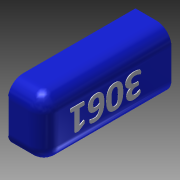
# Autodesk Inventor part: Bumper Cover Part4 (24x28 robot)
Saved by Autodesk Inventor 2013 (Build 170138000, 138)
## iProperties
Created: 2013-01-06
Part Number: Bumper Cover Part4 (24x28 robot)
Material: Generic
Document SubType Name: Modeling
Designer: Moses
Density: 1 g/cm^3
Mass: 165.217 g
Surface Area: 2027.83 cm^2
Volume: 165.217 cm^3
Author: Moses
Autodesk Inventor part; units mm, degrees
ref_plane "YZ Plane" through (0, 0, 0) normal (1, 0, 0) x (0, 1, 0)
ref_plane "XZ Plane" through (0, 0, 0) normal (0, 1, 0) x (-1, 0, 0)
ref_plane "XY Plane" through (0, 0, 0) normal (0, 0, 1) x (1, 0, 0)
sketch "Sketch1" plane through (0, 0, 0) normal (0, 0, 1) x (1, 0, 0)
  line L0 (-6.35, 63.5) -> (-6.35, -63.5) construction
  line L1 (6.35, 63.5) -> (-6.35, 63.5) construction
  line L2 (-6.35, -63.5) -> (6.35, -63.5) construction
  circle A0 centre (38.1, -31.75) radius 31.75 construction
  circle A1 centre (38.1, 31.75) radius 31.75 construction
  line L3 (6.35, 63.5) -> (38.1, 63.5) construction
  line L4 (69.85, 31.75) -> (69.85, -31.75) construction
  line L5 (6.35, -63.5) -> (38.1, -63.5) construction
  line L6 (38.1, 65.0875) -> (-7.9375, 65.0875)
  line L7 (-7.9375, -65.0875) -> (38.1, -65.0875)
  arc A2 (38.1, -65.0875) -> (71.4375, -31.75) centre (38.1, -31.75) ccw
  arc A3 (71.4375, 31.75) -> (38.1, 65.0875) centre (38.1, 31.75) ccw
  line L8 (71.4375, 31.75) -> (71.4375, -31.75)
  line L9 (38.1, 65.0875) -> (38.1, 63.5) construction
  arc A4 (69.85, 31.75) -> (38.1, 63.5) centre (38.1, 31.75) ccw
  arc A5 (38.1, -63.5) -> (69.85, -31.75) centre (38.1, -31.75) ccw
  line L10 (38.1, 63.5) -> (-6.35, 63.5)
  line L11 (38.1, -63.5) -> (-6.35, -63.5)
  line L12 (69.85, 31.75) -> (69.85, -31.75)
  line L13 (-6.35, 63.5) -> (-6.35, 38.1)
  line L14 (-6.35, 38.1) -> (-7.9375, 38.1)
  line L15 (-7.9375, 38.1) -> (-7.9375, 65.0875)
  line L16 (-7.9375, -65.0875) -> (-7.9375, -38.1)
  line L17 (-7.9375, -38.1) -> (-6.35, -38.1)
  line L18 (-6.35, -63.5) -> (-6.35, -38.1)
  line L19 (-6.35, 38.1) -> (-6.35, -38.1)
  point P0 (0, 0)
  point P1 (38.1, 64.2937)
  dimension "d3" = 25.4
  dimension "d5" = 1.5875
  dimension "d6" = 1.5875
  dimension "d7" = 25.4
  dimension "d9" = 1.5875
  constraints: 34 end point, 14 tangent, 12 point on circle, 6 perpendicular, 4 centre point, 3 collinear, 3 parallel, 2 coincident, 2 point on line, 1 concentric, 1 midpoint, 1 vertical
  measures "d3" distance of L0.start L13.end
  measures "d5" distance between parallel lines of L0 L15
  measures "d6" distance between parallel lines of L0 L16
  measures "d7" distance of L0.end L17.end
  measures "d9" distance of L6.start L3.end
extrude "Extrusion1" add sketch "Sketch1" along normal blind 1.5875
extrude "Extrusion2" add sketch "Sketch1" against normal blind 277.8125 contours A3 L8 A2 L7 L16 L17 L18 L11 A5 L12 A4 L10 L13 L14 L15 L6
sketch "Sketch2" plane through (0, 0, -277.8125) normal (0, 0, -1) x (-1, 0, 0)
  line L0 (-38.1, 63.5) -> (6.35, 63.5) projected
  line L1 (6.35, 63.5) -> (6.35, 38.1) projected
  line L2 (6.35, 38.1) -> (7.9375, 38.1) projected
  line L3 (7.9375, 38.1) -> (7.9375, 65.0875) projected
  line L4 (7.9375, 65.0875) -> (-38.1, 65.0875) projected
  arc A0 (-38.1, 65.0875) -> (-71.4375, 31.75) centre (-38.1, 31.75) ccw projected
  line L5 (-71.4375, 31.75) -> (-71.4375, -31.75) projected
  arc A1 (-71.4375, -31.75) -> (-38.1, -65.0875) centre (-38.1, -31.75) ccw projected
  line L6 (-38.1, -65.0875) -> (7.9375, -65.0875) projected
  line L7 (7.9375, -65.0875) -> (7.9375, -38.1) projected
  line L8 (7.9375, -38.1) -> (6.35, -38.1) projected
  line L9 (6.35, -38.1) -> (6.35, -63.5) projected
  line L10 (6.35, -63.5) -> (-38.1, -63.5) projected
  arc A2 (-69.85, -31.75) -> (-38.1, -63.5) centre (-38.1, -31.75) ccw projected
  line L11 (-69.85, -31.75) -> (-69.85, 31.75) projected
  arc A3 (-38.1, 63.5) -> (-69.85, 31.75) centre (-38.1, 31.75) ccw projected
  line L12 (6.35, 38.1) -> (6.35, -38.1)
  point P0 (0, 0)
  constraints: 2 end point, 1 parallel
extrude "Extrusion3" add sketch "Sketch2" along normal blind 1.5875
fillet "Fillet1" radius 33.3375 10 edges at (61.6732, -55.3232, 1.5875) (71.4375, 0, 1.5875) (61.6732, 55.3232, 1.5875) (15.0813, 65.0875, 1.5875) (15.0813, -65.0875, 1.5875) (60.5506, -54.2006, 0) (69.85, 0, 0) (60.5506, 54.2006, 0) (15.875, 63.5, 0) (15.875, -63.5, 0)
sketch "Sketch3" plane through (71.4375, -31.75, -279.4) normal (1, 0, 0) x (0, 0, -1)
  line L0 (-247.65, 0) -> (-247.65, 63.5) projected
  line L1 (0, 0) -> (-247.65, 0) projected
  line L2 (0, 63.5) -> (-247.65, 63.5) projected
  line L3 (-69.85, 0) -> (-222.25, 0) construction
  line L4 (-222.25, 0) -> (-222.25, 63.5) construction
  line L5 (-222.25, 63.5) -> (-69.85, 63.5) construction
  line L6 (-69.85, 63.5) -> (-69.85, 0) construction
  spline S0 degree 2 poles (-102.1187, 42.2439) (-102.1187, 46.0122) (-99.2091, 51.8792) (-94.0575, 55.886) (-86.8549, 57.937) (-82.6096, 57.937) knots 0 0 0 1 2 3 4 4 4
  spline S1 degree 2 poles (-82.6096, 57.937) (-80.0339, 57.937) (-75.5024, 57.1738) (-72.0203, 56.1245) (-69.7308, 54.932) (-69.063, 54.3119) (-68.6814, 53.501) (-68.3952, 52.4516) (-68.2998, 50.8775) (-68.2998, 49.7327) knots 0 0 0 1 2 3 4 5 6 7 8 8 8
  spline S2 degree 2 poles (-68.2998, 49.7327) (-68.2998, 47.8247) (-68.9199, 46.3938) (-69.54, 46.3938) knots 0 0 0 1 2 2 2
  spline S3 degree 2 poles (-69.54, 46.3938) (-69.9216, 46.3938) (-71.8772, 47.4431) (-74.8346, 48.6833) (-78.8414, 49.7327) (-81.3694, 49.7327) knots 0 0 0 1 2 3 4 4 4
  spline S4 degree 2 poles (-81.3694, 49.7327) (-83.5159, 49.7327) (-86.8072, 48.731) (-89.0968, 46.8707) (-90.2415, 44.2473) (-90.2415, 42.6732) knots 0 0 0 1 2 3 4 4 4
  spline S5 degree 2 poles (-90.2415, 42.6732) (-90.2415, 40.9083) (-88.8583, 38.094) (-86.1871, 36.0907) (-82.0849, 34.9936) (-79.2707, 34.9936) knots 0 0 0 1 2 3 4 4 4
  line L7 (-79.2707, 34.9936) -> (-74.8823, 34.9936)
  spline S6 degree 2 poles (-74.8823, 34.9936) (-74.4053, 34.9936) (-73.6898, 34.7074) (-73.2128, 33.8488) (-73.022, 32.3224) (-73.022, 31.1299) knots 0 0 0 1 2 3 4 4 4
  spline S7 degree 2 poles (-73.022, 31.1299) (-73.022, 29.9851) (-73.2128, 28.5541) (-73.6421, 27.7909) (-74.3099, 27.457) (-74.7869, 27.457) knots 0 0 0 1 2 3 4 4 4
  line L8 (-74.7869, 27.457) -> (-79.223, 27.457)
  spline S8 degree 2 poles (-79.223, 27.457) (-81.5125, 27.457) (-85.0423, 26.4077) (-87.4273, 24.452) (-88.6675, 21.6854) (-88.6675, 19.9682) knots 0 0 0 1 2 3 4 4 4
  spline S9 degree 2 poles (-88.6675, 19.9682) (-88.6675, 18.6803) (-87.8089, 16.3908) (-86.1394, 14.7213) (-83.4682, 13.7196) (-81.6556, 13.7196) knots 0 0 0 1 2 3 4 4 4
  spline S10 degree 2 poles (-81.6556, 13.7196) (-79.6046, 13.7196) (-76.0271, 14.9121) (-73.1651, 16.3908) (-71.1617, 17.6309) (-70.6847, 17.6309) knots 0 0 0 1 2 3 4 4 4
  spline S11 degree 2 poles (-70.6847, 17.6309) (-70.3985, 17.6309) (-69.9216, 17.3447) (-69.5877, 16.5815) (-69.4446, 15.1029) (-69.4446, 13.9104) knots 0 0 0 1 2 3 4 4 4
  spline S12 degree 2 poles (-69.4446, 13.9104) (-69.4446, 12.9564) (-69.54, 11.6685) (-69.7785, 10.8099) (-70.1123, 10.1898) (-70.8755, 9.4266) (-73.3082, 7.9479) (-76.9811, 6.5169) (-81.7987, 5.563) (-84.613, 5.563) knots 0 0 0 1 2 3 4 5 6 7 8 8 8
  spline S13 degree 2 poles (-84.613, 5.563) (-88.2859, 5.563) (-93.9621, 7.2801) (-97.8258, 10.5237) (-99.8292, 15.246) (-99.8292, 18.251) knots 0 0 0 1 2 3 4 4 4
  spline S14 degree 2 poles (-99.8292, 18.251) (-99.8292, 20.5406) (-98.6367, 24.4997) (-96.3948, 27.6478) (-92.9604, 29.842) (-90.7662, 30.3667) knots 0 0 0 1 2 3 4 4 4
  line L9 (-90.7662, 30.3667) -> (-90.7662, 30.5098)
  spline S15 degree 2 poles (-90.7662, 30.5098) (-93.3897, 30.796) (-97.635, 32.8948) (-100.5446, 35.9953) (-102.1187, 39.9543) (-102.1187, 42.2439) knots 0 0 0 1 2 3 4 4 4
  spline S16 degree 2 poles (-143.9035, 31.5592) (-143.9035, 37.617) (-141.9478, 47.3954) (-137.5118, 54.2642) (-130.4523, 57.937) (-125.3484, 57.937) knots 0 0 0 1 2 3 4 4 4
  spline S17 degree 2 poles (-125.3484, 57.937) (-120.1492, 57.937) (-113.3281, 54.3596) (-109.3691, 47.6816) (-107.7473, 38.0463) (-107.7473, 31.9408) knots 0 0 0 1 2 3 4 4 4
  spline S18 degree 2 poles (-107.7473, 31.9408) (-107.7473, 25.9307) (-109.7507, 16.1046) (-114.139, 9.2358) (-121.2462, 5.563) (-126.3024, 5.563) knots 0 0 0 1 2 3 4 4 4
  spline S19 degree 2 poles (-126.3024, 5.563) (-131.5016, 5.563) (-138.3704, 9.1404) (-142.3294, 15.8184) (-143.9035, 25.4537) (-143.9035, 31.5592) knots 0 0 0 1 2 3 4 4 4
  spline S20 degree 2 poles (-133.5527, 32.0362) (-133.5527, 28.4587) (-133.1711, 22.9256) (-132.3602, 18.8711) (-131.12, 16.0569) (-129.4029, 14.3874) (-127.2087, 13.6719) (-125.8731, 13.6719) knots 0 0 0 1 2 3 4 5 6 6 6
  spline S21 degree 2 poles (-125.8731, 13.6719) (-123.5835, 13.6719) (-120.5785, 15.9138) (-118.8136, 20.3498) (-118.0981, 27.0277) (-118.0981, 31.4161) knots 0 0 0 1 2 3 4 4 4
  spline S22 degree 2 poles (-118.0981, 31.4161) (-118.0981, 36.8538) (-118.9567, 43.9134) (-120.8169, 48.1109) (-123.6789, 49.7804) (-125.73, 49.7804) knots 0 0 0 1 2 3 4 4 4
  spline S23 degree 2 poles (-125.73, 49.7804) (-127.2564, 49.7804) (-129.5937, 48.7787) (-131.3585, 46.8231) (-132.551, 43.8657) (-133.2665, 39.9543) (-133.5527, 35.0413) (-133.5527, 32.0362) knots 0 0 0 1 2 3 4 5 6 6 6
  spline S24 degree 2 poles (-184.2096, 40.1451) (-184.2096, 43.9611) (-181.8723, 50.4959) (-177.3409, 55.2182) (-170.663, 57.937) (-166.3223, 57.937) knots 0 0 0 1 2 3 4 4 4
  spline S25 degree 2 poles (-166.3223, 57.937) (-162.8402, 57.937) (-157.5933, 56.3153) (-153.7773, 53.3102) (-151.3446, 49.0172) (-149.866, 43.6272) (-149.3413, 37.2831) (-149.3413, 33.7534) knots 0 0 0 1 2 3 4 5 6 6 6
  spline S26 degree 2 poles (-149.3413, 33.7534) (-149.3413, 30.796) (-149.9137, 24.3089) (-151.6308, 18.0602) (-154.6836, 12.384) (-159.4536, 8.091) (-166.3223, 5.6107) (-170.9969, 5.6107) knots 0 0 0 1 2 3 4 5 6 6 6
  spline S27 degree 2 poles (-170.9969, 5.6107) (-172.4755, 5.6107) (-175.5283, 5.9446) (-178.1041, 6.5169) (-179.869, 7.2324) (-180.4891, 7.7094) (-180.7753, 8.3295) (-180.9661, 9.0927) (-181.0615, 10.1898) (-181.0615, 10.953) knots 0 0 0 1 2 3 4 5 6 7 8 8 8
  spline S28 degree 2 poles (-181.0615, 10.953) (-181.0615, 12.1932) (-180.9661, 13.815) (-180.6322, 14.6736) (-180.0598, 15.1029) (-179.6782, 15.1029) knots 0 0 0 1 2 3 4 4 4
  spline S29 degree 2 poles (-179.6782, 15.1029) (-179.2012, 15.1029) (-177.7225, 14.5782) (-175.6237, 13.9581) (-172.7617, 13.4811) (-170.9015, 13.4811) knots 0 0 0 1 2 3 4 4 4
  spline S30 degree 2 poles (-170.9015, 13.4811) (-167.7056, 13.4811) (-163.3172, 15.8184) (-160.5984, 19.8251) (-159.3582, 25.1198) (-159.3105, 28.0771) knots 0 0 0 1 2 3 4 4 4
  spline S31 degree 2 poles (-159.3105, 28.0771) (-160.1691, 27.5524) (-162.4109, 26.4554) (-165.0344, 25.6922) (-168.0395, 25.1675) (-169.8044, 25.1675) knots 0 0 0 1 2 3 4 4 4
  spline S32 degree 2 poles (-169.8044, 25.1675) (-173.6203, 25.1675) (-179.1058, 27.2662) (-182.5878, 31.1776) (-184.2096, 36.7584) (-184.2096, 40.1451) knots 0 0 0 1 2 3 4 4 4
  spline S33 degree 2 poles (-174.145, 41.0991) (-174.145, 39.1434) (-173.4295, 36.0907) (-171.8554, 34.0396) (-169.2797, 32.9902) (-167.4671, 32.9902) knots 0 0 0 1 2 3 4 4 4
  spline S34 degree 2 poles (-167.4671, 32.9902) (-166.37, 32.9902) (-164.2235, 33.3718) (-162.2201, 34.0873) (-160.3122, 35.0413) (-159.5013, 35.6137) knots 0 0 0 1 2 3 4 4 4
  spline S35 degree 2 poles (-159.5013, 35.6137) (-159.5013, 39.7635) (-160.4553, 45.3921) (-162.2678, 48.6356) (-165.0821, 50.0189) (-166.8947, 50.0189) knots 0 0 0 1 2 3 4 4 4
  spline S36 degree 2 poles (-166.8947, 50.0189) (-168.7073, 50.0189) (-171.4261, 48.6833) (-173.191, 46.2507) (-174.145, 43.0071) (-174.145, 41.0991) knots 0 0 0 1 2 3 4 4 4
  spline S37 degree 2 poles (-223.514, 53.1194) (-223.514, 54.2165) (-223.2755, 55.7429) (-222.8462, 56.6492) (-222.3215, 57.0307) (-221.94, 57.0307) knots 0 0 0 1 2 3 4 4 4
  line L10 (-221.94, 57.0307) -> (-194.0357, 57.0307)
  spline S38 degree 2 poles (-194.0357, 57.0307) (-193.7018, 57.0307) (-193.1771, 56.6492) (-192.7478, 55.7429) (-192.5093, 54.2165) (-192.5093, 53.1194) knots 0 0 0 1 2 3 4 4 4
  spline S39 degree 2 poles (-192.5093, 53.1194) (-192.5093, 52.0223) (-192.7001, 50.4959) (-193.1294, 49.5419) (-193.7018, 49.1126) (-194.0357, 49.1126) knots 0 0 0 1 2 3 4 4 4
  line L11 (-194.0357, 49.1126) -> (-203.4325, 49.1126)
  line L12 (-203.4325, 49.1126) -> (-203.4325, 16.1523)
  line L13 (-203.4325, 16.1523) -> (-195.2759, 20.636)
  spline S40 degree 2 poles (-195.2759, 20.636) (-194.4173, 21.0653) (-193.2725, 21.2561) (-192.6047, 20.5883) (-192.3662, 18.9665) (-192.3662, 17.4878) knots 0 0 0 1 2 3 4 4 4
  spline S41 degree 2 poles (-192.3662, 17.4878) (-192.3662, 16.5338) (-192.4616, 15.3414) (-192.7478, 14.4828) (-193.3202, 13.9104) (-193.7972, 13.6242) knots 0 0 0 1 2 3 4 4 4
  line L14 (-193.7972, 13.6242) -> (-204.625, 6.6123)
  spline S42 degree 2 poles (-204.625, 6.6123) (-204.8635, 6.4215) (-205.4359, 6.2308) (-206.3899, 6.1354) (-207.9163, 6.0877) (-209.1088, 6.0877) knots 0 0 0 1 2 3 4 4 4
  spline S43 degree 2 poles (-209.1088, 6.0877) (-210.5875, 6.0877) (-212.4477, 6.1831) (-213.354, 6.4692) (-213.6879, 6.9462) (-213.6879, 7.2801) knots 0 0 0 1 2 3 4 4 4
  line L15 (-213.6879, 7.2801) -> (-213.6879, 49.1126)
  line L16 (-213.6879, 49.1126) -> (-221.94, 49.1126)
  spline S44 degree 2 poles (-221.94, 49.1126) (-222.3215, 49.1126) (-222.8939, 49.5419) (-223.3232, 50.4959) (-223.514, 52.0223) (-223.514, 53.1194) knots 0 0 0 1 2 3 4 4 4
  point P0 (-279.4, 31.75)
  dimension "d15" = 152.4
  dimension "d17" = 25.4
  constraints: 2 point on line, 2 other
  measures "d15" distance of L3.start L3.end
  measures "d17" distance between parallel lines of L0 L4
extrude "Extrusion4" add sketch "Sketch3" along normal blind 1.5875
body "Solid1"
